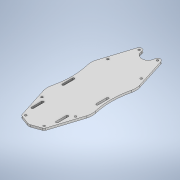
# Autodesk Inventor part: 399 prig top plate
Saved by Autodesk Inventor 2020 (Build 240168000, 168)
## iProperties
Created: 2022-05-23
Part Number: 399 prig top plate
Material: Generic
Document SubType Name: Modeling
Designer: Steven
Density: 1 g/cm^3
Appearance: Default
Author: Steven
Autodesk Inventor part; units mm, degrees
ref_plane "YZ Plane" through (0, 0, 0) normal (1, 0, 0) x (0, 1, 0)
ref_plane "XZ Plane" through (0, 0, 0) normal (0, 1, 0) x (-1, 0, 0)
ref_plane "XY Plane" through (0, 0, 0) normal (0, 0, 1) x (1, 0, 0)
sketch "Sketch1" plane through (0, 0, 0) normal (0, 1, 0) x (-1, 0, 0)
  arc A0 (23.1118, 83.4134) -> (26.1118, 83.4134) centre (24.6118, 83.4134) ccw
  line L0 (23.1118, 98.4134) -> (23.1118, 83.4134)
  arc A1 (26.1118, 98.4134) -> (23.1118, 98.4134) centre (24.6118, 98.4134) ccw
  line L1 (26.1118, 83.4134) -> (26.1118, 98.4134)
  arc A2 (16.2641, 134.7212) -> (19.2641, 134.7212) centre (17.7641, 134.7212) ccw
  line L2 (16.2641, 149.7212) -> (16.2641, 134.7212)
  arc A3 (19.2641, 149.7212) -> (16.2641, 149.7212) centre (17.7641, 149.7212) ccw
  line L3 (19.2641, 134.7212) -> (19.2641, 149.7212)
  arc A4 (-19.2641, 134.7212) -> (-16.2641, 134.7212) centre (-17.7641, 134.7212) ccw
  line L4 (-19.2641, 149.7212) -> (-19.2641, 134.7212)
  arc A5 (-16.2641, 149.7212) -> (-19.2641, 149.7212) centre (-17.7641, 149.7212) ccw
  line L5 (-16.2641, 134.7212) -> (-16.2641, 149.7212)
  arc A6 (-26.1118, 83.4134) -> (-23.1118, 83.4134) centre (-24.6118, 83.4134) ccw
  line L6 (-26.1118, 98.4134) -> (-26.1118, 83.4134)
  arc A7 (-23.1118, 98.4134) -> (-26.1118, 98.4134) centre (-24.6118, 98.4134) ccw
  line L7 (-23.1118, 83.4134) -> (-23.1118, 98.4134)
  circle A8 centre (-24.2029, 34.3759) radius 1.5
  circle A9 centre (-13.2835, 163.8268) radius 1.5
  circle A10 centre (24.2029, 129.4508) radius 1.5
  circle A11 centre (13.2835, 0) radius 1.5
  arc A12 (-31.7205, 55.8278) -> (-31.7205, 107.999) centre (-139.6118, 81.9134) ccw
  arc A13 (-31.7205, 55.8278) -> (-31.2853, 43.4596) centre (-9.3646, 50.4227) ccw
  line L8 (-31.2853, 43.4596) -> (-17.0958, -1.211)
  arc A14 (-17.0958, -1.211) -> (-9.2835, 0) centre (-13.2835, 0) ccw
  arc A15 (9.2835, 0) -> (-9.2835, 0) centre (0, 0) ccw
  arc A16 (9.2835, 0) -> (17.0958, -1.211) centre (13.2835, 0) ccw
  line L9 (17.0958, -1.211) -> (31.2853, 43.4596)
  arc A17 (31.2853, 43.4596) -> (31.7205, 55.8278) centre (9.3646, 50.4227) ccw
  arc A18 (31.7205, 107.999) -> (31.7205, 55.8278) centre (139.6118, 81.9134) ccw
  arc A19 (31.7205, 107.999) -> (31.2853, 120.3671) centre (9.3646, 113.4041) ccw
  line L10 (31.2853, 120.3671) -> (17.0958, 165.0377)
  arc A20 (17.0958, 165.0377) -> (14.6505, 167.5859) centre (13.2835, 163.8268) ccw
  line L11 (14.6505, 167.5859) -> (2.0505, 172.1678)
  arc A21 (2.0505, 172.1678) -> (-2.0505, 172.1678) centre (0, 166.529) ccw
  line L12 (-2.0505, 172.1678) -> (-14.6505, 167.5859)
  arc A22 (-14.6505, 167.5859) -> (-17.0958, 165.0377) centre (-13.2835, 163.8268) ccw
  line L13 (-17.0958, 165.0377) -> (-31.2853, 120.3671)
  arc A23 (-31.2853, 120.3671) -> (-31.7205, 107.999) centre (-9.3646, 113.4041) ccw
  circle A24 centre (24.2029, 34.3759) radius 1.5
  circle A25 centre (13.2835, 163.8268) radius 1.5
  circle A26 centre (-24.2029, 129.4508) radius 1.5
  circle A27 centre (-13.2835, 0) radius 1.5
  point P0 (31.7205, 107.999)
  point P1 (31.2853, 120.3671)
  point P2 (17.0958, 165.0377)
  point P3 (14.6505, 167.5859)
  point P4 (-31.7205, 55.8278)
  point P5 (-31.2853, 43.4596)
  point P6 (-17.0958, -1.211)
  point P7 (-9.2835, 0)
  point P8 (9.2835, 0)
  point P9 (31.7205, 55.8278)
  point P10 (19.2641, 149.7212)
  point P11 (16.2641, 149.7212)
  point P12 (23.1118, 98.4134)
  constraints: 40 point on circle, 28 centre point, 28 end point
extrude "Extrusion1" add sketch "Sketch1" along normal blind 3
body "Solid1"
